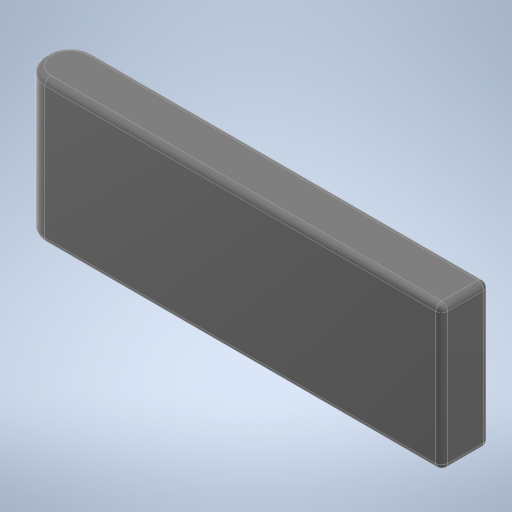
# Autodesk Inventor part: Lipo-3250-3S-Pack-3
Saved by Autodesk Inventor 2024.2 (Build 282272000, 272)
## iProperties
Created: 2024-01-26
Part Number: Lipo-3250-3S-Pack-3
Material: Acetal Resin, Black
Document SubType Name: Modeling
Designer: Masato Kubotera
Mass: 249 g
Surface Area: 184.876 cm^2
Volume: 105.762 cm^3
Density: 2.35434 g/cm^3
Appearance: Smooth - Black
Catalog Web Link: https://maxamps.com/products/lipo-2800-3s-11-1v-battery-pack
Vendor: MaxAmps
Author: Masato Kubotera
Autodesk Inventor part; units mm, degrees
ref_plane "YZ Plane" through (0, 0, 0) normal (1, 0, 0) x (0, 1, 0)
ref_plane "XZ Plane" through (0, 0, 0) normal (0, 1, 0) x (-1, 0, 0)
ref_plane "XY Plane" through (0, 0, 0) normal (0, 0, 1) x (1, 0, 0)
sketch "Sketch1" plane through (0, 0, 0) normal (0, 0, 1) x (1, 0, 0)
  line L0 (-8, -70) -> (8, -70)
  line L1 (8, -70) -> (8, 70)
  line L2 (8, 70) -> (-8, 70)
  line L3 (-8, 70) -> (-8, -70)
  line L4 (-8, -70) -> (8, 70) construction
  line L5 (8, -70) -> (-8, 70) construction
  point P0 (0, 0)
  dimension "d0" = 16
  dimension "d1" = 140
  constraints: 12 end point, 2 midpoint, 2 parallel, 1 horizontal, 1 perpendicular
  measures "d0" distance of L1.end L2.end
  measures "d1" distance of L0.end L1.end
extrude "Extrusion1" add sketch "Sketch1" along normal blind 48
fillet "Fillet1" radius 2 10 edges at (8, 70, 24) (-8, 70, 24) (0, 70, 48) (8, 0, 48) (-8, 0, 48) (8, 0, 0) (0, 70, 0) (-8, 0, 0) (0, -70, 48) (0, -70, 0)
fillet "Fillet2" radius 7.5 6 edges at (7.4142, -69.4142, 47.4142) (7.4142, -69.4142, 0.5858) (8, -70, 24) (-7.4142, -69.4142, 47.4142) (-7.4142, -69.4142, 0.5858) (-8, -70, 24)
body "Solid1"
